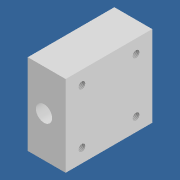
# Autodesk Inventor part: Linear_Unit_B
Saved by Autodesk Inventor 2020 (Build 240168000, 168)
## iProperties
Created: 2021-07-13
Part Number: Linear_Unit_B
Material: 一般
Document SubType Name: Modeling
Designer: ken113
Density: 1 g/cm^3
Appearance: 既定
Author: ken113
Autodesk Inventor part; units mm, degrees
ref_plane "YZ Plane" through (0, 0, 0) normal (1, 0, 0) x (0, 1, 0)
ref_plane "XZ Plane" through (0, 0, 0) normal (0, 1, 0) x (-1, 0, 0)
ref_plane "XY Plane" through (0, 0, 0) normal (0, 0, 1) x (1, 0, 0)
sketch "スケッチ1" plane through (0, 0, 0) normal (1, 0, 0) x (0, 1, 0)
  line L0 (-15, -16) -> (15, -16)
  line L1 (15, -16) -> (15, 16)
  line L2 (15, 16) -> (-15, 16)
  line L3 (-15, 16) -> (-15, -16)
  line L4 (-15, -16) -> (15, 16) construction
  line L5 (15, -16) -> (-15, 16) construction
  point P0 (0, 0)
  dimension "d0" = 32
  dimension "d1" = 30
  constraints: 12 end point, 2 midpoint, 2 parallel, 1 horizontal, 1 perpendicular
  measures "d0" distance of L0.end L1.end
  measures "d1" distance of L1.end L2.end
extrude "押し出し1" add sketch "スケッチ1" along normal blind 14
sketch "スケッチ2" plane through (0, -15, 16) normal (0, 0, 1) x (1, 0, 0)
  line L0 (0, 30) -> (0, 0) projected
  line L1 (0, 0) -> (14, 0) projected
  line L2 (14, 30) -> (14, 0) projected
  line L3 (0, 30) -> (14, 30) projected
  circle A0 centre (6, 15) radius 3
  point P0 (0, 15)
  dimension "d4" = 6
  dimension "d17" = 6
  constraints: 1 centre point, 1 coincident
  measures "d4" diameter of A0
  measures "d17" distance from line of A0.centre L0
extrude "押し出し2" cut sketch "スケッチ2" against normal through all contours A0
sketch "スケッチ3" plane through (14, 0, 0) normal (1, 0, 0) x (0, 0, -1)
  line L0 (-10, 10) -> (10, 10)
  line L1 (10, 10) -> (10, -10)
  line L2 (10, -10) -> (-10, -10)
  line L3 (-10, -10) -> (-10, 10)
  line L4 (-10, 10) -> (10, -10) construction
  line L5 (10, 10) -> (-10, -10) construction
  line L6 (-16, 15) -> (-16, -15) projected
  point P0 (0, 0)
  point P1 (0, 0)
  dimension "d7" = 20
  dimension "d8" = 20
  dimension "d9" = 6
  constraints: 12 end point, 2 midpoint, 2 parallel, 1 horizontal, 1 perpendicular
  measures "d7" distance of L1.end L2.end
  measures "d8" distance of L0.end L1.end
  measures "d9" distance between parallel lines of L3 L6
hole "穴1" at (14, 10, -10) at (14, 10, 10) at (14, -10, 10) at (14, -10, -10) direction (-1, 0, 0) diameter 2.459 depth 8.8 thread size "M3x0.5" class "6H" standard "ISO Metric profile"
